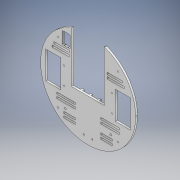
# Autodesk Inventor part: LBase
Saved by Autodesk Inventor 2017 (Build 210142000, 142)
## iProperties
Part Number: LBase
Material: Genérico
Document SubType Name: Modeling
Designer: Roberto
Density: 1 g/cm^3
Appearance: Valor por defecto
Author: Roberto
Autodesk Inventor part; units mm, degrees
ref_plane "YZ Plane" through (0, 0, 0) normal (1, 0, 0) x (0, 1, 0)
ref_plane "XZ Plane" through (0, 0, 0) normal (0, 1, 0) x (-1, 0, 0)
ref_plane "XY Plane" through (0, 0, 0) normal (0, 0, 1) x (1, 0, 0)
sketch "Boceto1" plane through (0, 0, 0) normal (0, 1, 0) x (-1, 0, 0)
  line L0 (4.925, -3.9) -> (4.925, -4.2)
  line L1 (4.925, -4.2) -> (2.025, -4.2)
  line L2 (2.025, -4.2) -> (2.025, -3.9)
  line L3 (2.025, -3.9) -> (4.925, -3.9)
  line L4 (-4.925, -3.3) -> (-2.025, -3.3)
  line L5 (-2.025, -3.3) -> (-2.025, -3.6)
  line L6 (-2.025, -3.6) -> (-4.925, -3.6)
  line L7 (-4.925, -3.6) -> (-4.925, -3.3)
  line L8 (3, 2.4695) -> (3, 2.7695)
  line L9 (3, 2.7695) -> (5.7, 2.7695)
  line L10 (5.7, 2.7695) -> (5.7, 2.4695)
  line L11 (5.7, 2.4695) -> (3, 2.4695)
  line L12 (3, 3.0695) -> (3, 3.3695)
  line L13 (3, 3.3695) -> (5.4, 3.3695)
  line L14 (5.4, 3.3695) -> (5.4, 3.0695)
  line L15 (5.4, 3.0695) -> (3, 3.0695)
  line L16 (2.025, -5.4) -> (3.825, -5.4)
  line L17 (3.825, -5.4) -> (3.825, -5.7)
  line L18 (3.825, -5.7) -> (2.025, -5.7)
  line L19 (2.025, -5.7) -> (2.025, -5.4)
  line L20 (-3.825, -5.7) -> (-3.825, -5.4)
  line L21 (-3.825, -5.4) -> (-2.025, -5.4)
  line L22 (-2.025, -5.4) -> (-2.025, -5.7)
  line L23 (-2.025, -5.7) -> (-3.825, -5.7)
  line L24 (-3.825, -6.3) -> (-3.825, -6)
  line L25 (-3.825, -6) -> (-2.025, -6)
  line L26 (-2.025, -6) -> (-2.025, -6.3)
  line L27 (-2.025, -6.3) -> (-3.825, -6.3)
  line L28 (2.025, -6.3) -> (2.025, -6)
  line L29 (2.025, -6) -> (3.825, -6)
  line L30 (3.825, -6) -> (3.825, -6.3)
  line L31 (3.825, -6.3) -> (2.025, -6.3)
  line L32 (-3, 3.3695) -> (-3, 3.0695)
  line L33 (-3, 3.0695) -> (-5.4, 3.0695)
  line L34 (-5.4, 3.0695) -> (-5.4, 3.3695)
  line L35 (-5.4, 3.3695) -> (-3, 3.3695)
  line L36 (-3, 2.7695) -> (-3, 2.4695)
  line L37 (-3, 2.4695) -> (-5.7, 2.4695)
  line L38 (-5.7, 2.4695) -> (-5.7, 2.7695)
  line L39 (-5.7, 2.7695) -> (-3, 2.7695)
  line L40 (-4.925, -4.2) -> (-4.925, -3.9)
  line L41 (-4.925, -3.9) -> (-2.025, -3.9)
  line L42 (-2.025, -3.9) -> (-2.025, -4.2)
  line L43 (-2.025, -4.2) -> (-4.925, -4.2)
  line L44 (4.925, -3.6) -> (2.025, -3.6)
  line L45 (2.025, -3.6) -> (2.025, -3.3)
  line L46 (2.025, -3.3) -> (4.925, -3.3)
  line L47 (4.925, -3.3) -> (4.925, -3.6)
  line L48 (0.15, -6.5) -> (-0.15, -6.5)
  line L49 (-1.2, -6.5) -> (-1.5, -6.5)
  line L50 (1.5, -6.5) -> (1.2, -6.5)
  line L51 (-6.725, -2.7) -> (-6.725, 1.7)
  line L52 (-6.725, 1.7) -> (-4.325, 1.7)
  line L53 (-4.325, 1.7) -> (-4.325, -2.7)
  line L54 (-4.325, -2.7) -> (-6.725, -2.7)
  line L55 (4.3, -2.7) -> (4.3, 1.7)
  line L56 (4.3, 1.7) -> (6.7, 1.7)
  line L57 (6.7, 1.7) -> (6.7, -2.7)
  line L58 (6.7, -2.7) -> (4.3, -2.7)
  circle A0 centre (-4.734, 4.334) radius 0.1
  circle A1 centre (4.734, 4.334) radius 0.1
  circle A2 centre (-4.734, -5.334) radius 0.1
  circle A3 centre (4.734, -5.334) radius 0.1
  circle A4 centre (-3.8, 0.894) radius 0.1
  circle A5 centre (-3.8, -1.894) radius 0.1
  circle A6 centre (3.8, 0.894) radius 0.1
  circle A7 centre (3.8, -1.894) radius 0.1
  line L59 (2.55, -1.4) -> (-2.55, -1.4)
  line L60 (1.5, -1.4) -> (1.5, -6.5)
  line L61 (1.2, -6.5) -> (1.2, -1.4)
  line L62 (0.15, -1.4) -> (0.15, -6.5)
  line L63 (-0.15, -6.5) -> (-0.15, -1.4)
  line L64 (-1.5, -6.5) -> (-1.5, -1.4)
  line L65 (-1.2, -1.4) -> (-1.2, -6.5)
  line L66 (2.55, -1.4) -> (2.55, 6.6532)
  line L67 (-2.55, -1.4) -> (-2.55, 6.6532)
  line L68 (-7.5, -0.5) -> (-7.5, -0.4)
  line L69 (7.5, -0.5) -> (7.5, -0.4)
  line L70 (-7.5, -0.5) -> (-7.5, -0.6)
  line L71 (7.4993, -0.5) -> (7.4993, -0.6)
  arc A8 (-7.5, -0.6) -> (7.4993, -0.6) centre (-0.0003, -0.6) ccw
  arc A9 (7.4993, -0.5) -> (2.55, 6.6532) centre (0, -0.4) ccw
  arc A10 (-2.55, 6.6532) -> (-7.5, -0.4) centre (0, -0.4) ccw
  line L72 (-4.734, -5.184) -> (-5.4457, -5.184)
  line L73 (-4.734, -5.234) -> (-4.734, -5.334)
  point P0 (2.352, 6.909)
  dimension "d43" = 0.2
  dimension "d13" = 0.1
  dimension "d14" = 0.1
  dimension "d15" = 0.1
  dimension "d39" = 0.2
  dimension "d40" = 0.2
  dimension "d41" = 0.2
  dimension "d42" = 0.2
  dimension "d44" = 0.2
  dimension "d45" = 0.2
  dimension "d46" = 0.2
  constraints: 148 end point, 10 centre point, 7 point on line, 6 point on circle, 5 vertical, 1 horizontal, 1 tangent, 1 vertical alignment, 2 other
  measures "d13" distance of L68.end L68.start
  measures "d14" distance of L69.start L69.end
  measures "d15" distance of L68.start L70.end
  measures "d39" diameter of A1
  measures "d40" diameter of A6
  measures "d41" diameter of A7
  measures "d42" diameter of A3
  measures "d44" diameter of A0
  measures "d45" diameter of A4
  measures "d46" diameter of A5
extrude "Extrusión1" add sketch "Boceto1" along normal blind 0.3 contours L62 L59 L61 L50 L60 L66 A9 L69 L71 A8 L70 L68 A10 L67 L64 L49 L65 L63 L48
sketch "Boceto2" plane through (0, 0.3, 0) normal (0, 1, 0) x (1, 0, 0)
  line L0 (-1.2, 6.5) -> (-1.2, 1.4) projected
  line L1 (-1.5, 1.4) -> (-1.5, 6.5) projected
  line L2 (-0.15, 1.4) -> (-0.15, 6.5) projected
  line L3 (0.15, 6.5) -> (0.15, 1.4) projected
  line L4 (1.2, 1.4) -> (1.2, 6.5) projected
  line L5 (1.5, 6.5) -> (1.5, 1.4) projected
  line L6 (1.2, 6.5) -> (1.5, 6.5) projected
  line L7 (-0.15, 6.5) -> (0.15, 6.5) projected
  line L8 (-1.5, 6.5) -> (-1.2, 6.5) projected
  line L9 (-1.5, 6.5) -> (-1.2, 6.5)
  line L10 (-1.2, 6.5) -> (-1.2, 1.4)
  line L11 (-1.2, 1.4) -> (-1.5, 1.4)
  line L12 (-1.5, 1.4) -> (-1.5, 6.5)
  line L13 (-0.15, 6.5) -> (0.15, 6.5)
  line L14 (0.15, 6.5) -> (0.15, 1.4)
  line L15 (0.15, 1.4) -> (-0.15, 1.4)
  line L16 (-0.15, 1.4) -> (-0.15, 6.5)
  line L17 (1.2, 6.5) -> (1.5, 6.5)
  line L18 (1.5, 6.5) -> (1.5, 1.4)
  line L19 (1.5, 1.4) -> (1.2, 1.4)
  line L20 (1.2, 1.4) -> (1.2, 6.5)
  point P0 (0, 0)
  constraints: 24 end point, 6 parallel, 3 horizontal, 3 perpendicular
extrude "Extrusión2" add sketch "Boceto2" along normal mid plane 0.6
sketch "Boceto3" plane through (-2.4, 0, -1.4) normal (0, 0, 1) x (1, 0, 0)
  line L0 (0, 0) -> (4.8, 0)
  line L1 (0, 0.3) -> (4.8, 0.3)
  line L2 (0, 0.3) -> (4.8, 0.3)
  line L3 (9.9, 0.3) -> (-5.1, 0.3)
  line L4 (4.8, 0) -> (0, 0)
  line L5 (9.9, 0) -> (-5.1, 0)
  line L6 (-0.3, 0.15) -> (-0.15, 0)
  line L7 (-0.3, 0.15) -> (-0.15, 0.3)
  line L8 (5.1, 0.15) -> (4.95, 0.3)
  line L9 (5.1, 0.15) -> (4.95, 0)
  line L10 (-0.15, 0.3) -> (4.95, 0.3)
  line L11 (4.95, 0) -> (-0.15, 0)
  point P0 (2.4, 0)
  point P1 (0.048, 0)
  point P2 (4.752, 0)
  constraints: 24 end point, 3 collinear, 1 point on line
extrude "Extrusión3" cut sketch "Boceto3" along normal blind 10
sketch "Boceto4" plane through (0, 0.3, 0) normal (0, 1, 0) x (1, 0, 0)
  circle A0 centre (-0.675, 7) radius 0.15
  line L0 (4.325, -1.7) -> (4.325, 2.7)
  circle A1 centre (0.675, 7) radius 0.15
  line L1 (-6.7, -1.7) -> (-6.7, 2.7)
  line L2 (-6.7, 2.7) -> (-4.3, 2.7)
  line L3 (-4.3, 2.7) -> (-4.3, -1.7)
  line L4 (-4.3, -1.7) -> (-6.7, -1.7)
  line L5 (4.325, 2.7) -> (6.725, 2.7)
  line L6 (6.725, 2.7) -> (6.725, -1.7)
  line L7 (-3.825, 5.8) -> (-2.025, 5.8)
  line L8 (-2.025, 5.5) -> (-3.825, 5.5)
  line L9 (2.025, 5.8) -> (3.825, 5.8)
  line L10 (3.825, 5.5) -> (2.025, 5.5)
  line L11 (4.325, 2.7) -> (6.725, 2.7) projected
  line L12 (2.025, 6.3) -> (3.825, 6.3) projected
  circle A2 centre (-0.675, 7) radius 0.1
  circle A3 centre (0.675, 7) radius 0.1
  point P0 (0, 0)
  dimension "d47" = 0.3
  dimension "d48" = 0.2
  dimension "d49" = 0.2
  constraints: 22 end point, 4 centre point, 2 coincident
  measures "d47" diameter of A0
  measures "d48" diameter of A2
  measures "d49" diameter of A3
extrude "Extrusión4" cut sketch "Boceto4" against normal blind 10 contours A2 | A3
sketch "Boceto8" plane through (0, 0.3, 0) normal (0, 1, 0) x (1, 0, 0)
  circle A0 centre (-3.8, -0.894) radius 0.1 projected
  line L0 (0, 0) -> (0, -2.4412)
  circle A1 centre (3.8, -0.894) radius 0.1
  circle A2 centre (3.6, 4.906) radius 0.15
  circle A3 centre (-3.6, 4.906) radius 0.15
  dimension "d33" = 0.3
  dimension "d34" = 0.3
  constraints: 3 centre point, 2 end point, 1 symmetric about line, 1 vertical, 1 other
  measures "d33" diameter of A2
  measures "d34" diameter of A3
extrude "Extrusión6" cut sketch "Boceto8" against normal blind 10 contours A2 | A3
sketch "Boceto9" plane through (0, 0, 0) normal (0, -1, 0) x (1, 0, 0)
  line L0 (-2.85, 3.6695) -> (-4.09, 3.6695)
  line L1 (-4.09, 5.5295) -> (-4.09, 3.6695)
  line L2 (-2.85, 3.6695) -> (-2.85, 5.5295)
  line L3 (-4.09, 5.5295) -> (-2.85, 5.5295)
  line L4 (-3, 3.3695) -> (-5.4, 3.3695) projected
  line L5 (-2.55, 6.6532) -> (-2.55, -1.4) projected
  point P0 (0, 0)
  constraints: 8 end point, 2 vertical
extrude "Extrusión7" cut sketch "Boceto9" against normal blind 10
sketch "Boceto11" plane through (0, 0, 0) normal (0, -1, 0) x (1, 0, 0)
  line L0 (-2.85, 5.5295) -> (-4.09, 5.5295) projected
  line L1 (-2.85, 5.5295) -> (-3.15, 5.5295)
  line L2 (-3.15, 5.5295) -> (-3.15, 5.5795)
  line L3 (-4.09, 5.5295) -> (-3.79, 5.5295)
  line L4 (-3.79, 5.5295) -> (-3.79, 5.5795)
  line L5 (-3.79, 5.5795) -> (-3.15, 5.5795)
  line L6 (-4.09, 5.5295) -> (-4.09, 3.6695)
  line L7 (-4.09, 3.6695) -> (-4.09, 5.5295) projected
  line L8 (-2.85, 3.6695) -> (-3.15, 3.6695)
  line L9 (-3.15, 3.6695) -> (-3.15, 3.6195)
  line L10 (-4.09, 3.6695) -> (-3.79, 3.6695)
  line L11 (-3.79, 3.6695) -> (-3.79, 3.6195)
  line L12 (-3.79, 3.6195) -> (-3.15, 3.6195)
  line L13 (-2.85, 5.5295) -> (-2.85, 3.6695)
  point P0 (0, 0)
  dimension "d50" = 0.3
  dimension "d51" = 0.05
  dimension "d52" = 0.3
  dimension "d53" = 0.05
  constraints: 24 end point, 2 perpendicular, 2 point on line, 2 vertical
  measures "d50" distance of L0.start L1.end
  measures "d51" distance of L1.end L2.end
  measures "d52" distance of L0.end L3.end
  measures "d53" distance of L3.end L4.end
extrude "Extrusión8" cut sketch "Boceto11" against normal blind 10
